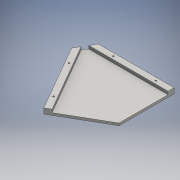
# Autodesk Inventor part: bottom half
Saved by Autodesk Inventor 2016 SP1 (Build 200210100, 210)
## iProperties
Created: 2016-04-14
Part Number: bottom half
Material: Generic
Document SubType Name: Modeling
Designer: ubik
Density: 1 g/cm^3
Appearance: Default
Author: ubik
Autodesk Inventor part; units mm, degrees
ref_plane "YZ Plane" through (0, 0, 0) normal (1, 0, 0) x (0, 1, 0)
ref_plane "XZ Plane" through (0, 0, 0) normal (0, 1, 0) x (-1, 0, 0)
ref_plane "XY Plane" through (0, 0, 0) normal (0, 0, 1) x (1, 0, 0)
sketch "Sketch1" plane through (0, 0, 0) normal (0, 0, 1) x (1, 0, 0)
  line L0 (-32.2735, -28.2023) -> (32.2735, -28.2023) projected
  line L1 (32.2735, -28.2023) -> (282.2736, 404.8104) projected
  line L2 (282.2736, 404.8104) -> (250.0001, 460.7098) projected
  line L3 (250.0001, 460.7098) -> (-249.9999, 460.71) projected
  line L4 (-249.9999, 460.71) -> (-282.2735, 404.8106) projected
  line L5 (-282.2735, 404.8106) -> (-32.2735, -28.2023) projected
  line L6 (0, -28.2023) -> (0, 279.1061)
  line L7 (-266.1368, 432.7601) -> (0, 279.1059)
  line L8 (266.1368, 432.7601) -> (0, 279.1061)
  line L9 (0, 279.1061) -> (0.0001, 460.7099)
  line L10 (0, 279.1061) -> (-157.2735, 188.3042)
  line L11 (0, 279.1059) -> (157.2736, 188.3041)
  point P0 (0, 0)
  constraints: 12 end point, 6 midpoint, 1 point on line
extrude "Extrusion1" add sketch "Sketch1" along normal blind 18 contours L5 L4 L7 L10 | L7 L4 L3 L9
sketch "Sketch2" plane through (0, 0, 18) normal (0, 0, 1) x (1, 0, 0)
  line L0 (0, 279.1059) -> (0.0001, 460.7099) projected
  line L1 (0.0001, 460.7099) -> (-249.9999, 460.71) projected
  line L2 (-249.9999, 460.71) -> (-282.2735, 404.8106) projected
  line L3 (-282.2735, 404.8106) -> (-157.2735, 188.3042) projected
  line L4 (-157.2735, 188.3042) -> (0, 279.106) projected
  line L5 (0, 279.1059) -> (0, 279.106) projected
  line L6 (-261.5469, 440.71) -> (0.0001, 440.7099)
  line L7 (-139.953, 198.3042) -> (-270.7265, 424.8106)
  point P0 (0, 0)
  dimension "d2" = 20
  constraints: 4 end point, 4 point on line
  measures "d2" distance between parallel lines of L1 L6
extrude "Extrusion2" cut sketch "Sketch2" against normal blind 10 contours L4 L7 L2 L6 L0
sketch "Sketch3" plane through (0, 0, 18) normal (0, 0, 1) x (1, 0, 0)
  circle A0 centre (-189.9999, 450.71) radius 2.5
  circle A1 centre (-49.9999, 450.7099) radius 2.5
  circle A2 centre (-243.6132, 357.849) radius 2.5
  circle A3 centre (-173.6132, 236.6055) radius 2.5
  line L0 (0.0001, 460.7099) -> (-249.9999, 460.71) projected
  line L1 (0.0001, 440.7099) -> (0.0001, 460.7099) projected
  line L2 (-282.2735, 404.8106) -> (-157.2735, 188.3042) projected
  line L3 (-157.2735, 188.3042) -> (-139.953, 198.3042) projected
  point P0 (0, 0)
  dimension "d5" = 5
  dimension "d6" = 5
  dimension "d7" = 5
  dimension "d8" = 5
  dimension "d9" = 10
  dimension "d10" = 10
  dimension "d11" = 50
  dimension "d12" = 190
  dimension "d13" = 10
  dimension "d14" = 10
  dimension "d15" = 50
  dimension "d16" = 190
  constraints: 4 centre point
  measures "d5" diameter of A0
  measures "d6" diameter of A1
  measures "d7" diameter of A2
  measures "d8" diameter of A3
  measures "d9" distance from line of L0 A0.centre
  measures "d10" distance from line of L0 A1.centre
  measures "d11" distance from line of L1 A1.centre
  measures "d12" distance from line of L1 A0.centre
  measures "d13" distance from line of L2 A3.centre
  measures "d14" distance from line of L2 A2.centre
  measures "d15" distance from line of L3 A3.centre
  measures "d16" distance from line of L3 A2.centre
extrude "Extrusion3" cut sketch "Sketch3" against normal through all
equation "\"d10\" = d9"
equation "\"d13\" = d9"
equation "\"d14\" = d9"
equation "\"d15\" = d11"
equation "\"d16\" = d12"
body "Solid1"
